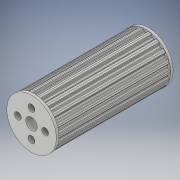
# Autodesk Inventor part: Pulley
Saved by Autodesk Inventor 2019 (Build 230136000, 136)
## iProperties
Created: 2019-03-22
Part Number: Pulley
Material: Generic
Document SubType Name: Modeling
Designer: frown
Density: 1 g/cm^3
Appearance: Default
Author: frown
Autodesk Inventor part; units mm, degrees
ref_plane "YZ Plane" through (0, 0, 0) normal (1, 0, 0) x (0, 1, 0)
ref_plane "XZ Plane" through (0, 0, 0) normal (0, 1, 0) x (-1, 0, 0)
ref_plane "XY Plane" through (0, 0, 0) normal (0, 0, 1) x (1, 0, 0)
sketch "Sketch1" plane through (-11.8161, 5.8463, 20) normal (0, 0, 1) x (1, 0, 0)
  circle A0 centre (11.8162, -5.8464) radius 2.6001 projected
  line L0 (0.3323, 2.2358) -> (0.845, 1.4636) construction
  line L1 (2.7121, 3.6888) -> (1.8626, 4.0596)
  line L2 (0.8623, 3.345) -> (1.4764, 4.0152)
  line L3 (0.8623, 3.345) -> (0.309, 2.6238)
  line L4 (0.3323, 2.2358) -> (0.845, 1.4636)
  line L5 (3.8664, 4.3699) -> (3.1355, 3.7567)
  arc A1 (1.8626, 4.0596) -> (1.4764, 4.0152) centre (1.7083, 3.7) ccw
  arc A2 (2.7121, 3.6888) -> (3.1355, 3.7567) centre (2.8686, 4.0672) ccw
  arc A3 (0.309, 2.6238) -> (0.3323, 2.2358) centre (0.6547, 2.4499) ccw
  arc A4 (0.8516, 1.0348) -> (0.845, 1.4636) centre (0.4997, 1.2438) ccw
  arc A5 (-0.8406, -3.1302) -> (-0.9935, -2.7296) centre (-1.2428, -3.0542) ccw
  line L6 (-1.7394, -2.1793) -> (-0.9935, -2.7296)
  line L7 (0, 0) -> (-0.9251, 0.0579)
  arc A6 (-1.894, -1.8227) -> (-1.7394, -2.1793) centre (-1.5096, -1.8679) ccw
  arc A7 (-0.9251, 0.0579) -> (-1.2729, -0.1159) centre (-0.9471, -0.3328) ccw
  line L8 (-1.6207, -0.9557) -> (-1.894, -1.8227)
  line L9 (-1.6207, -0.9557) -> (-1.2729, -0.1159)
  arc A8 (-1.0063, -7.6229) -> (-1.287, -7.2987) centre (-1.4102, -7.689) ccw
  line L10 (-0.8406, -3.1302) -> (-1.0063, -4.0697)
  arc A9 (-1.287, -4.3939) -> (-1.0063, -4.0697) centre (-1.4103, -4.0035) ccw
  line L11 (-2.1761, -7.0367) -> (-1.287, -7.2987)
  line L12 (-1.287, -4.3939) -> (-2.1761, -4.6559)
  arc A10 (-2.4433, -6.7544) -> (-2.1761, -7.0367) centre (-2.0667, -6.6655) ccw
  arc A11 (-2.1761, -4.6559) -> (-2.4434, -4.9382) centre (-2.0631, -5.0306) ccw
  line L13 (-2.4831, -5.8463) -> (-2.4433, -6.7544)
  line L14 (-2.4831, -5.8463) -> (-2.4434, -4.9382)
  arc A12 (0.3746, -11.9013) -> (0, -11.6926) centre (0.0177, -12.1015) ccw
  line L15 (-1.0063, -7.6229) -> (-0.8406, -8.5624)
  arc A13 (-0.9935, -8.963) -> (-0.8406, -8.5624) centre (-1.243, -8.6384) ccw
  line L16 (-0.9251, -11.7505) -> (0, -11.6926)
  line L17 (-0.9935, -8.963) -> (-1.7394, -9.5133)
  arc A14 (-1.2728, -11.5767) -> (-0.9251, -11.7505) centre (-0.9493, -11.3643) ccw
  arc A15 (-1.7394, -9.5133) -> (-1.8941, -9.87) centre (-1.5051, -9.8268) ccw
  line L18 (-1.6207, -10.7369) -> (-1.2728, -11.5767)
  line L19 (-1.6207, -10.7369) -> (-1.8941, -9.87)
  arc A16 (3.1356, -15.4493) -> (2.7121, -15.3814) centre (2.8686, -15.7595) ccw
  line L20 (0.3746, -11.9013) -> (0.8516, -12.7274)
  arc A17 (0.845, -13.1562) -> (0.8516, -12.7274) centre (0.4995, -12.9364) ccw
  line L21 (1.8627, -15.7522) -> (2.7121, -15.3814)
  line L22 (0.845, -13.1562) -> (0.3323, -13.9284)
  arc A18 (1.4765, -15.7078) -> (1.8627, -15.7522) centre (1.7078, -15.3975) ccw
  arc A19 (0.3323, -13.9284) -> (0.309, -14.3165) centre (0.6597, -14.1428) ccw
  line L23 (0.8623, -15.0376) -> (1.4765, -15.7078)
  line L24 (0.8623, -15.0376) -> (0.309, -14.3165)
  arc A20 (6.9435, -17.8391) -> (6.5224, -17.9201) centre (6.7988, -18.2219) ccw
  line L25 (3.1356, -15.4493) -> (3.8663, -16.0625)
  arc A21 (4.0068, -16.4677) -> (3.8663, -16.0625) centre (3.607, -16.3793) ccw
  line L26 (5.8509, -18.5591) -> (6.5224, -17.9201)
  line L27 (4.0068, -16.4677) -> (3.7891, -17.3687)
  arc A22 (5.4728, -18.6494) -> (5.8509, -18.5591) centre (5.5841, -18.2787) ccw
  arc A23 (3.7891, -17.3687) -> (3.8999, -17.7413) centre (4.1701, -17.4582) ccw
  line L28 (4.6665, -18.2297) -> (5.4728, -18.6494)
  line L29 (4.6665, -18.2297) -> (3.8999, -17.7413)
  arc A24 (11.3391, -18.7824) -> (10.9711, -19.0025) centre (11.3341, -19.1916) ccw
  line L30 (6.9435, -17.8391) -> (7.8399, -18.1654)
  arc A25 (8.1105, -18.4981) -> (7.8399, -18.1654) centre (7.7046, -18.5518) ccw
  line L31 (10.5587, -19.8326) -> (10.9711, -19.0025)
  line L32 (8.1105, -18.4981) -> (8.2141, -19.4192)
  arc A26 (10.2343, -20.0468) -> (10.5587, -19.8326) centre (10.2121, -19.6604) ccw
  arc A27 (8.2141, -19.4192) -> (8.4456, -19.7315) centre (8.6027, -19.373) ccw
  line L33 (9.3331, -19.9282) -> (10.2343, -20.0468)
  line L34 (9.3331, -19.9282) -> (8.4456, -19.7315)
  arc A28 (15.7923, -18.1654) -> (15.5217, -18.4981) centre (15.9275, -18.5517) ccw
  line L35 (11.3391, -18.7824) -> (12.2931, -18.7824)
  arc A29 (12.6611, -19.0025) -> (12.2931, -18.7824) centre (12.2981, -19.1918) ccw
  line L36 (15.4181, -19.4192) -> (15.5217, -18.4981)
  line L37 (12.6611, -19.0025) -> (13.0735, -19.8326)
  arc A30 (15.1866, -19.7314) -> (15.4181, -19.4192) centre (15.0335, -19.3759) ccw
  arc A31 (13.0735, -19.8326) -> (13.3979, -20.0469) centre (13.4229, -19.6563) ccw
  line L38 (14.2991, -19.9282) -> (15.1866, -19.7314)
  line L39 (14.2991, -19.9282) -> (13.3979, -20.0469)
  arc A32 (19.7658, -16.0625) -> (19.6254, -16.4677) centre (20.025, -16.3793) ccw
  line L40 (15.7923, -18.1654) -> (16.6887, -17.8391)
  arc A33 (17.1098, -17.9201) -> (16.6887, -17.8391) centre (16.8334, -18.2221) ccw
  line L41 (19.8431, -17.3687) -> (19.6254, -16.4677)
  line L42 (17.1098, -17.9201) -> (17.7813, -18.5591)
  arc A34 (19.7323, -17.7413) -> (19.8431, -17.3687) centre (19.4669, -17.4596) ccw
  arc A35 (17.7813, -18.5591) -> (18.1594, -18.6495) centre (18.0493, -18.2739) ccw
  line L43 (18.9657, -18.2297) -> (19.7323, -17.7413)
  line L44 (18.9657, -18.2297) -> (18.1594, -18.6495)
  arc A36 (22.7806, -12.7274) -> (22.7872, -13.1562) centre (23.1325, -12.9364) ccw
  line L45 (19.7658, -16.0625) -> (20.4967, -15.4493)
  arc A37 (20.9201, -15.3814) -> (20.4967, -15.4493) centre (20.7636, -15.7598) ccw
  line L46 (23.2999, -13.9284) -> (22.7872, -13.1562)
  line L47 (20.9201, -15.3814) -> (21.7695, -15.7522)
  arc A38 (23.3232, -14.3164) -> (23.2999, -13.9284) centre (22.9775, -14.1425) ccw
  arc A39 (21.7695, -15.7522) -> (22.1558, -15.7078) centre (21.9239, -15.3926) ccw
  line L48 (22.7699, -15.0376) -> (23.3232, -14.3164)
  line L49 (22.7699, -15.0376) -> (22.1558, -15.7078)
  arc A40 (24.4728, -8.5624) -> (24.6257, -8.963) centre (24.875, -8.6384) ccw
  line L50 (22.7806, -12.7274) -> (23.2576, -11.9012)
  arc A41 (23.6322, -11.6926) -> (23.2576, -11.9012) centre (23.6146, -12.1017) ccw
  line L51 (25.3716, -9.5133) -> (24.6257, -8.963)
  line L52 (23.6322, -11.6926) -> (24.5573, -11.7505)
  arc A42 (25.5262, -9.8699) -> (25.3716, -9.5133) centre (25.1418, -9.8247) ccw
  arc A43 (24.5573, -11.7505) -> (24.9051, -11.5767) centre (24.5793, -11.3598) ccw
  line L53 (25.2529, -10.7369) -> (25.5262, -9.8699)
  line L54 (25.2529, -10.7369) -> (24.9051, -11.5767)
  arc A44 (24.6385, -4.0697) -> (24.9192, -4.3939) centre (25.0424, -4.0036) ccw
  line L55 (24.4728, -8.5624) -> (24.6385, -7.6229)
  arc A45 (24.9192, -7.2987) -> (24.6385, -7.6229) centre (25.0425, -7.6891) ccw
  line L56 (25.8083, -4.6559) -> (24.9192, -4.3939)
  line L57 (24.9192, -7.2987) -> (25.8083, -7.0367)
  arc A46 (26.0755, -4.9382) -> (25.8083, -4.6559) centre (25.6989, -5.0271) ccw
  arc A47 (25.8083, -7.0367) -> (26.0756, -6.7544) centre (25.6953, -6.662) ccw
  line L58 (26.1153, -5.8463) -> (26.0755, -4.9382)
  line L59 (26.1153, -5.8463) -> (26.0756, -6.7544)
  arc A48 (23.2576, 0.2087) -> (23.6322, 0) centre (23.6145, 0.4089) ccw
  line L60 (24.6385, -4.0697) -> (24.4728, -3.1302)
  arc A49 (24.6257, -2.7296) -> (24.4728, -3.1302) centre (24.8752, -3.0542) ccw
  line L61 (24.5573, 0.0579) -> (23.6322, 0)
  line L62 (24.6257, -2.7296) -> (25.3716, -2.1793)
  arc A50 (24.905, -0.1159) -> (24.5573, 0.0579) centre (24.5815, -0.3283) ccw
  arc A51 (25.3716, -2.1793) -> (25.5263, -1.8226) centre (25.1373, -1.8658) ccw
  line L63 (25.2529, -0.9557) -> (24.905, -0.1159)
  line L64 (25.2529, -0.9557) -> (25.5263, -1.8226)
  arc A52 (20.4966, 3.7567) -> (20.9201, 3.6888) centre (20.7636, 4.0669) ccw
  line L65 (23.2576, 0.2087) -> (22.7806, 1.0348)
  arc A53 (22.7872, 1.4636) -> (22.7806, 1.0348) centre (23.1327, 1.2438) ccw
  line L66 (21.7695, 4.0596) -> (20.9201, 3.6888)
  line L67 (22.7872, 1.4636) -> (23.2999, 2.2358)
  arc A54 (22.1557, 4.0152) -> (21.7695, 4.0596) centre (21.9244, 3.7049) ccw
  arc A55 (23.2999, 2.2358) -> (23.3232, 2.6239) centre (22.9725, 2.4502) ccw
  line L68 (22.7699, 3.345) -> (22.1557, 4.0152)
  line L69 (22.7699, 3.345) -> (23.3232, 2.6239)
  arc A56 (16.6887, 6.1465) -> (17.1098, 6.2275) centre (16.8334, 6.5293) ccw
  line L70 (20.4966, 3.7567) -> (19.7659, 4.3699)
  arc A57 (19.6254, 4.7751) -> (19.7659, 4.3699) centre (20.0252, 4.6867) ccw
  line L71 (17.7813, 6.8665) -> (17.1098, 6.2275)
  line L72 (19.6254, 4.7751) -> (19.8431, 5.6761)
  arc A58 (18.1594, 6.9568) -> (17.7813, 6.8665) centre (18.0481, 6.5861) ccw
  arc A59 (19.8431, 5.6761) -> (19.7323, 6.0487) centre (19.4621, 5.7656) ccw
  line L73 (18.9657, 6.5371) -> (18.1594, 6.9568)
  line L74 (18.9657, 6.5371) -> (19.7323, 6.0487)
  arc A60 (12.2931, 7.0898) -> (12.6611, 7.3099) centre (12.2981, 7.499) ccw
  line L75 (16.6887, 6.1465) -> (15.7923, 6.4728)
  arc A61 (15.5217, 6.8055) -> (15.7923, 6.4728) centre (15.9276, 6.8592) ccw
  line L76 (13.0735, 8.14) -> (12.6611, 7.3099)
  line L77 (15.5217, 6.8055) -> (15.4181, 7.7266)
  arc A62 (13.3979, 8.3542) -> (13.0735, 8.14) centre (13.4201, 7.9678) ccw
  arc A63 (15.4181, 7.7266) -> (15.1866, 8.0389) centre (15.0295, 7.6804) ccw
  line L78 (14.2991, 8.2356) -> (13.3979, 8.3542)
  line L79 (14.2991, 8.2356) -> (15.1866, 8.0389)
  arc A64 (7.8399, 6.4728) -> (8.1105, 6.8055) centre (7.7047, 6.8591) ccw
  line L80 (12.2931, 7.0898) -> (11.3391, 7.0898)
  arc A65 (10.9711, 7.3099) -> (11.3391, 7.0898) centre (11.3341, 7.4992) ccw
  line L81 (8.2141, 7.7266) -> (8.1105, 6.8055)
  line L82 (10.9711, 7.3099) -> (10.5587, 8.14)
  arc A66 (8.4456, 8.0388) -> (8.2141, 7.7266) centre (8.5987, 7.6833) ccw
  arc A67 (10.5587, 8.14) -> (10.2343, 8.3543) centre (10.2093, 7.9637) ccw
  line L83 (9.3331, 8.2356) -> (8.4456, 8.0388)
  line L84 (9.3331, 8.2356) -> (10.2343, 8.3543)
  arc A68 (3.8664, 4.3699) -> (4.0068, 4.7751) centre (3.6072, 4.6867) ccw
  line L85 (7.8399, 6.4728) -> (6.9435, 6.1465)
  arc A69 (6.5224, 6.2275) -> (6.9435, 6.1465) centre (6.7988, 6.5295) ccw
  line L86 (3.7891, 5.6761) -> (4.0068, 4.7751)
  line L87 (6.5224, 6.2275) -> (5.8509, 6.8665)
  arc A70 (3.8999, 6.0487) -> (3.7891, 5.6761) centre (4.1653, 5.767) ccw
  arc A71 (5.8509, 6.8665) -> (5.4728, 6.9569) centre (5.5829, 6.5813) ccw
  line L88 (4.6665, 6.5371) -> (3.8999, 6.0487)
  line L89 (4.6665, 6.5371) -> (5.4728, 6.9569)
  line L90 (0.8516, 1.0348) -> (0.3746, 0.2087)
  arc A72 (0, 0) -> (0.3746, 0.2087) centre (0.0176, 0.4092) ccw
  point P0 (11.8161, -5.8463)
  point P1 (0.2852, 2.3363)
  point P2 (2.819, 3.66)
  point P3 (2.9298, 3.6623)
  point P4 (1.6446, 4.0861)
  point P5 (0.9089, 1.2538)
  point P6 (20.4966, 3.7567)
  point P7 (16.6887, 6.1465)
  point P8 (12.2931, 7.0898)
  point P9 (7.8399, 6.4728)
  point P10 (-0.8617, -2.9048)
  point P11 (0.2136, 0.0496)
  point P12 (-1.1391, 0.0082)
  point P13 (-1.1032, -7.4183)
  point P14 (-1.1032, -4.2743)
  point P15 (-2.3601, -4.7758)
  point P16 (0.2136, -11.7421)
  point P17 (-0.8617, -8.7877)
  point P18 (-1.8714, -9.6889)
  point P19 (2.9298, -15.3549)
  point P20 (0.9089, -12.9464)
  point P21 (0.2683, -14.1385)
  point P22 (6.7179, -17.8207)
  point P23 (3.995, -16.2487)
  point P24 (3.8009, -17.588)
  point P25 (11.1208, -18.8423)
  point P26 (8.0245, -18.2964)
  point P27 (8.3001, -19.6213)
  point P28 (15.6076, -18.2963)
  point P29 (12.5114, -18.8423)
  point P30 (13.2235, -19.9931)
  point P31 (19.6371, -16.2487)
  point P32 (16.9143, -17.8208)
  point P33 (17.9771, -18.6586)
  point P34 (22.7233, -12.9464)
  point P35 (20.7024, -15.3549)
  point P36 (21.9876, -15.7787)
  point P37 (24.4939, -8.7878)
  point P38 (23.4186, -11.7422)
  point P39 (24.7713, -11.7008)
  point P40 (24.7354, -4.2743)
  point P41 (24.7354, -7.4183)
  point P42 (25.9923, -6.9168)
  point P43 (23.4186, 0.0495)
  point P44 (24.4939, -2.9049)
  point P45 (25.5036, -2.0037)
  point P46 (20.7024, 3.6623)
  point P47 (22.7233, 1.2538)
  point P48 (23.3639, 2.4459)
  point P49 (16.9143, 6.1281)
  point P50 (19.6372, 4.5561)
  point P51 (19.8313, 5.8954)
  point P52 (20.4966, 3.7567)
  point P53 (12.5114, 7.1497)
  point P54 (15.6077, 6.6038)
  point P55 (15.3321, 7.9287)
  point P56 (16.6887, 6.1465)
  point P57 (8.0246, 6.6037)
  point P58 (11.1208, 7.1497)
  point P59 (10.4087, 8.3005)
  point P60 (12.2931, 7.0898)
  point P61 (3.9951, 4.5561)
  point P62 (6.7179, 6.1282)
  point P63 (5.6551, 6.966)
  point P64 (7.8399, 6.4728)
  dimension "d2" = 360
  constraints: 198 point on circle, 180 end point, 72 centre point, 34 coincident, 1 collinear, 1 tangent, 19 other
sketch "Sketch2" plane through (-11.8161, 5.8463, 20) normal (0, 0, 1) x (1, 0, 0)
  line L0 (0.8623, 3.345) -> (0.309, 2.6238) projected
  line L1 (1.4764, 4.0152) -> (0.8623, 3.345) projected
  line L2 (2.7121, 3.6888) -> (1.8626, 4.0596) projected
  line L3 (0.3323, 2.2358) -> (0.845, 1.4636) projected
  arc A0 (2.7121, 3.6888) -> (3.1355, 3.7567) centre (2.8686, 4.0672) ccw
  arc A1 (1.8626, 4.0596) -> (1.4764, 4.0152) centre (1.7083, 3.7) ccw
  arc A2 (0.309, 2.6238) -> (0.3323, 2.2358) centre (0.6591, 2.4501) ccw
  arc A3 (0.8516, 1.0348) -> (0.845, 1.4636) centre (0.4999, 1.2439) ccw
  line L4 (0.8516, 1.0348) -> (11.8161, -5.8463)
  line L5 (11.8161, -5.8463) -> (3.1355, 3.7567)
  point P0 (1.6446, 4.0861)
  point P1 (0.9089, 1.2538)
  point P2 (2.9298, 3.6623)
  point P3 (2.9298, 3.6623)
  point P4 (0.2683, 2.4458)
  point P5 (0.2683, 2.4458)
  constraints: 12 point on circle, 4 centre point, 4 end point, 2 coincident
extrude "Extrusion1" add sketch "Sketch2" along normal blind 0.125
pattern_circular "Circular Pattern1" count 18 over 360 about axis through (0, 0, 20) along (0, 0, 1) of "Extrusion1"
sketch "Sketch3" plane through (-11.8161, 5.8463, 20.125) normal (0, 0, 1) x (1, 0, 0)
  line L0 (11.8161, -5.8463) -> (3.1355, 3.7567) projected
  line L1 (3.8663, 4.3699) -> (11.8161, -5.8463) projected
  line L2 (3.1355, 3.7567) -> (3.8663, 4.3699)
  constraints: 2 end point
extrude "Extrusion2" add sketch "Sketch3" against normal blind 0.125
pattern_circular "Circular Pattern2" count 18 over 360 about axis through (0, 0, 20) along (0, 0, 1) of "Extrusion2"
sketch "Sketch4" plane through (-11.8161, 5.8463, 20.125) normal (0, 0, 1) x (1, 0, 0)
  arc A0 (6.5224, 6.2275) -> (6.9435, 6.1465) centre (6.7988, 6.5295) ccw projected
  line L0 (6.5224, 6.2275) -> (5.8509, 6.8665) projected
  arc A1 (5.8509, 6.8665) -> (5.4728, 6.9569) centre (5.5829, 6.5813) ccw projected
  line L1 (5.4728, 6.9569) -> (4.6665, 6.5371) projected
  line L2 (4.6665, 6.5371) -> (3.8999, 6.0487) projected
  arc A2 (3.8999, 6.0487) -> (3.7891, 5.6761) centre (4.1695, 5.7657) ccw projected
  line L3 (3.7891, 5.6761) -> (4.0068, 4.7751) projected
  arc A3 (3.8663, 4.3699) -> (4.0068, 4.7751) centre (3.6073, 4.6866) ccw projected
  line L4 (3.1355, 3.7567) -> (3.8663, 4.3699) projected
  arc A4 (2.7121, 3.6888) -> (3.1355, 3.7567) centre (2.8686, 4.0672) ccw projected
  line L5 (2.7121, 3.6888) -> (1.8626, 4.0596) projected
  arc A5 (1.8626, 4.0596) -> (1.4764, 4.0152) centre (1.7083, 3.7) ccw projected
  line L6 (1.4764, 4.0152) -> (0.8623, 3.345) projected
  line L7 (0.8623, 3.345) -> (0.309, 2.6238) projected
  arc A6 (0.309, 2.6238) -> (0.3323, 2.2358) centre (0.6591, 2.4501) ccw projected
  line L8 (0.3323, 2.2358) -> (0.845, 1.4636) projected
  arc A7 (0.8516, 1.0348) -> (0.845, 1.4636) centre (0.4999, 1.2439) ccw projected
  line L9 (0.3746, 0.2086) -> (0.8516, 1.0348) projected
  arc A8 (0, 0) -> (0.3746, 0.2086) centre (0.0176, 0.4091) ccw projected
  line L10 (0, 0) -> (-0.9251, 0.0579) projected
  arc A9 (-0.9251, 0.0579) -> (-1.2729, -0.1159) centre (-0.9471, -0.3328) ccw projected
  line L11 (-1.2729, -0.1159) -> (-1.6207, -0.9557) projected
  line L12 (-1.6207, -0.9557) -> (-1.894, -1.8227) projected
  arc A10 (-1.894, -1.8227) -> (-1.7394, -2.1793) centre (-1.5056, -1.8661) ccw projected
  line L13 (-1.7394, -2.1793) -> (-0.9935, -2.7296) projected
  arc A11 (-0.8407, -3.1302) -> (-0.9935, -2.7296) centre (-1.2426, -3.0541) ccw projected
  line L14 (-1.0063, -4.0697) -> (-0.8407, -3.1302) projected
  arc A12 (-1.287, -4.3939) -> (-1.0063, -4.0697) centre (-1.4103, -4.0035) ccw projected
  line L15 (-1.287, -4.3939) -> (-2.1761, -4.6559) projected
  arc A13 (-2.1761, -4.6559) -> (-2.4434, -4.9382) centre (-2.0631, -5.0306) ccw projected
  line L16 (-2.4434, -4.9382) -> (-2.4831, -5.8463) projected
  line L17 (-2.4831, -5.8463) -> (-2.4433, -6.7544) projected
  arc A14 (-2.4433, -6.7544) -> (-2.1761, -7.0367) centre (-2.0635, -6.6625) ccw projected
  line L18 (-2.1761, -7.0367) -> (-1.287, -7.2987) projected
  arc A15 (-1.0063, -7.6229) -> (-1.287, -7.2987) centre (-1.4101, -7.6888) ccw projected
  line L19 (-0.8406, -8.5624) -> (-1.0063, -7.6229) projected
  arc A16 (-0.9935, -8.963) -> (-0.8406, -8.5624) centre (-1.243, -8.6384) ccw projected
  line L20 (-0.9935, -8.963) -> (-1.7394, -9.5133) projected
  arc A17 (-1.7394, -9.5133) -> (-1.8941, -9.87) centre (-1.5051, -9.8268) ccw projected
  line L21 (-1.8941, -9.87) -> (-1.6207, -10.7369) projected
  line L22 (-1.6207, -10.7369) -> (-1.2728, -11.5767) projected
  arc A18 (-1.2728, -11.5767) -> (-0.9251, -11.7505) centre (-0.9473, -11.3604) ccw projected
  line L23 (-0.9251, -11.7505) -> (0, -11.6926) projected
  arc A19 (0.3746, -11.9013) -> (0, -11.6926) centre (0.0177, -12.1013) ccw projected
  line L24 (0.8516, -12.7274) -> (0.3746, -11.9013) projected
  arc A20 (0.845, -13.1562) -> (0.8516, -12.7274) centre (0.4995, -12.9364) ccw projected
  line L25 (0.845, -13.1562) -> (0.3323, -13.9284) projected
  arc A21 (0.3323, -13.9284) -> (0.309, -14.3165) centre (0.6597, -14.1428) ccw projected
  line L26 (0.309, -14.3165) -> (0.8623, -15.0376) projected
  line L27 (0.8623, -15.0376) -> (1.4765, -15.7078) projected
  arc A22 (1.4765, -15.7078) -> (1.8627, -15.7522) centre (1.7083, -15.3932) ccw projected
  line L28 (1.8627, -15.7522) -> (2.7121, -15.3814) projected
  arc A23 (3.1355, -15.4493) -> (2.7121, -15.3814) centre (2.8686, -15.7594) ccw projected
  line L29 (3.8663, -16.0625) -> (3.1355, -15.4493) projected
  arc A24 (4.0068, -16.4677) -> (3.8663, -16.0625) centre (3.607, -16.3793) ccw projected
  line L30 (4.0068, -16.4677) -> (3.7891, -17.3687) projected
  arc A25 (3.7891, -17.3687) -> (3.8999, -17.7413) centre (4.1701, -17.4582) ccw projected
  line L31 (3.8999, -17.7413) -> (4.6665, -18.2297) projected
  line L32 (4.6665, -18.2297) -> (5.4728, -18.6494) projected
  arc A26 (5.4728, -18.6494) -> (5.8509, -18.5591) centre (5.5831, -18.2745) ccw projected
  line L33 (5.8509, -18.5591) -> (6.5224, -17.9201) projected
  arc A27 (6.9435, -17.8391) -> (6.5224, -17.9201) centre (6.7987, -18.2218) ccw projected
  line L34 (7.8399, -18.1654) -> (6.9435, -17.8391) projected
  arc A28 (8.1105, -18.4981) -> (7.8399, -18.1654) centre (7.7046, -18.5518) ccw projected
  line L35 (8.1105, -18.4981) -> (8.2141, -19.4192) projected
  arc A29 (8.2141, -19.4192) -> (8.4456, -19.7315) centre (8.6027, -19.373) ccw projected
  line L36 (8.4456, -19.7315) -> (9.3331, -19.9282) projected
  line L37 (9.3331, -19.9282) -> (10.2343, -20.0468) projected
  arc A30 (10.2343, -20.0468) -> (10.5587, -19.8326) centre (10.2097, -19.6568) ccw projected
  line L38 (10.5587, -19.8326) -> (10.9711, -19.0025) projected
  arc A31 (11.3391, -18.7824) -> (10.9711, -19.0025) centre (11.3339, -19.1915) ccw projected
  line L39 (12.2931, -18.7824) -> (11.3391, -18.7824) projected
  arc A32 (12.6611, -19.0025) -> (12.2931, -18.7824) centre (12.2981, -19.1918) ccw projected
  line L40 (12.6611, -19.0025) -> (13.0735, -19.8326) projected
  arc A33 (13.0735, -19.8326) -> (13.3979, -20.0469) centre (13.4229, -19.6563) ccw projected
  line L41 (13.3979, -20.0469) -> (14.2991, -19.9282) projected
  line L42 (14.2991, -19.9282) -> (15.1866, -19.7314) projected
  arc A34 (15.1866, -19.7314) -> (15.4181, -19.4192) centre (15.0301, -19.3733) ccw projected
  line L43 (15.4181, -19.4192) -> (15.5217, -18.4981) projected
  arc A35 (15.7923, -18.1654) -> (15.5217, -18.4981) centre (15.9273, -18.5516) ccw projected
  line L44 (16.6887, -17.8391) -> (15.7923, -18.1654) projected
  arc A36 (17.1098, -17.9201) -> (16.6887, -17.8391) centre (16.8334, -18.2221) ccw projected
  line L45 (17.1098, -17.9201) -> (17.7813, -18.5591) projected
  arc A37 (17.7813, -18.5591) -> (18.1594, -18.6495) centre (18.0493, -18.2739) ccw projected
  line L46 (18.1594, -18.6495) -> (18.9657, -18.2297) projected
  line L47 (18.9657, -18.2297) -> (19.7323, -17.7413) projected
  arc A38 (19.7323, -17.7413) -> (19.8431, -17.3687) centre (19.4627, -17.4583) ccw projected
  line L48 (19.8431, -17.3687) -> (19.6254, -16.4677) projected
  arc A39 (19.7659, -16.0625) -> (19.6254, -16.4677) centre (20.0249, -16.3792) ccw projected
  line L49 (20.4967, -15.4493) -> (19.7659, -16.0625) projected
  arc A40 (20.9201, -15.3814) -> (20.4967, -15.4493) centre (20.7636, -15.7598) ccw projected
  line L50 (20.9201, -15.3814) -> (21.7695, -15.7522) projected
  arc A41 (21.7695, -15.7522) -> (22.1558, -15.7078) centre (21.9239, -15.3926) ccw projected
  line L51 (22.1558, -15.7078) -> (22.7699, -15.0376) projected
  line L52 (22.7699, -15.0376) -> (23.3232, -14.3164) projected
  arc A42 (23.3232, -14.3164) -> (23.2999, -13.9284) centre (22.9731, -14.1427) ccw projected
  line L53 (23.2999, -13.9284) -> (22.7872, -13.1562) projected
  arc A43 (22.7806, -12.7275) -> (22.7872, -13.1562) centre (23.1323, -12.9365) ccw projected
  line L54 (23.2576, -11.9012) -> (22.7806, -12.7275) projected
  arc A44 (23.6322, -11.6926) -> (23.2576, -11.9012) centre (23.6146, -12.1017) ccw projected
  line L55 (23.6322, -11.6926) -> (24.5573, -11.7505) projected
  arc A45 (24.5573, -11.7505) -> (24.9051, -11.5767) centre (24.5793, -11.3598) ccw projected
  line L56 (24.9051, -11.5767) -> (25.2529, -10.7369) projected
  line L57 (25.2529, -10.7369) -> (25.5262, -9.8699) projected
  arc A46 (25.5262, -9.8699) -> (25.3716, -9.5133) centre (25.1378, -9.8265) ccw projected
  line L58 (25.3716, -9.5133) -> (24.6257, -8.963) projected
  arc A47 (24.4729, -8.5624) -> (24.6257, -8.963) centre (24.8748, -8.6385) ccw projected
  line L59 (24.6385, -7.6229) -> (24.4729, -8.5624) projected
  arc A48 (24.9192, -7.2987) -> (24.6385, -7.6229) centre (25.0425, -7.6891) ccw projected
  line L60 (24.9192, -7.2987) -> (25.8083, -7.0367) projected
  arc A49 (25.8083, -7.0367) -> (26.0756, -6.7544) centre (25.6953, -6.662) ccw projected
  line L61 (26.0756, -6.7544) -> (26.1153, -5.8463) projected
  line L62 (26.1153, -5.8463) -> (26.0755, -4.9382) projected
  arc A50 (26.0755, -4.9382) -> (25.8083, -4.6559) centre (25.6957, -5.0301) ccw projected
  line L63 (25.8083, -4.6559) -> (24.9192, -4.3939) projected
  arc A51 (24.6385, -4.0697) -> (24.9192, -4.3939) centre (25.0423, -4.0038) ccw projected
  line L64 (24.4728, -3.1302) -> (24.6385, -4.0697) projected
  arc A52 (24.6257, -2.7296) -> (24.4728, -3.1302) centre (24.8752, -3.0542) ccw projected
  line L65 (24.6257, -2.7296) -> (25.3716, -2.1793) projected
  arc A53 (25.3716, -2.1793) -> (25.5263, -1.8226) centre (25.1373, -1.8658) ccw projected
  line L66 (25.5263, -1.8226) -> (25.2529, -0.9557) projected
  line L67 (25.2529, -0.9557) -> (24.905, -0.1159) projected
  arc A54 (24.905, -0.1159) -> (24.5573, 0.0579) centre (24.5795, -0.3322) ccw projected
  line L68 (24.5573, 0.0579) -> (23.6322, 0) projected
  arc A55 (23.2576, 0.2087) -> (23.6322, 0) centre (23.6145, 0.4087) ccw projected
  line L69 (22.7806, 1.0348) -> (23.2576, 0.2087) projected
  arc A56 (22.7872, 1.4636) -> (22.7806, 1.0348) centre (23.1327, 1.2438) ccw projected
  line L70 (22.7872, 1.4636) -> (23.2999, 2.2358) projected
  arc A57 (23.2999, 2.2358) -> (23.3232, 2.6239) centre (22.9725, 2.4502) ccw projected
  line L71 (23.3232, 2.6239) -> (22.7699, 3.345) projected
  line L72 (22.7699, 3.345) -> (22.1557, 4.0152) projected
  arc A58 (22.1557, 4.0152) -> (21.7695, 4.0596) centre (21.9239, 3.7006) ccw projected
  line L73 (21.7695, 4.0596) -> (20.9201, 3.6888) projected
  arc A59 (20.4967, 3.7567) -> (20.9201, 3.6888) centre (20.7636, 4.0668) ccw projected
  line L74 (19.7659, 4.3699) -> (20.4967, 3.7567) projected
  arc A60 (19.6254, 4.7751) -> (19.7659, 4.3699) centre (20.0252, 4.6867) ccw projected
  line L75 (19.6254, 4.7751) -> (19.8431, 5.6761) projected
  arc A61 (19.8431, 5.6761) -> (19.7323, 6.0487) centre (19.4621, 5.7656) ccw projected
  line L76 (19.7323, 6.0487) -> (18.9657, 6.5371) projected
  line L77 (18.9657, 6.5371) -> (18.1594, 6.9568) projected
  arc A62 (18.1594, 6.9568) -> (17.7813, 6.8665) centre (18.0491, 6.5819) ccw projected
  line L78 (17.7813, 6.8665) -> (17.1098, 6.2275) projected
  arc A63 (16.6887, 6.1465) -> (17.1098, 6.2275) centre (16.8335, 6.5292) ccw projected
  line L79 (15.7923, 6.4728) -> (16.6887, 6.1465) projected
  arc A64 (15.5217, 6.8055) -> (15.7923, 6.4728) centre (15.9276, 6.8592) ccw projected
  line L80 (15.5217, 6.8055) -> (15.4181, 7.7266) projected
  arc A65 (15.4181, 7.7266) -> (15.1866, 8.0389) centre (15.0295, 7.6804) ccw projected
  line L81 (15.1866, 8.0389) -> (14.2991, 8.2356) projected
  line L82 (14.2991, 8.2356) -> (13.3979, 8.3542) projected
  arc A66 (13.3979, 8.3542) -> (13.0735, 8.14) centre (13.4225, 7.9642) ccw projected
  line L83 (13.0735, 8.14) -> (12.6611, 7.3099) projected
  arc A67 (12.2931, 7.0898) -> (12.6611, 7.3099) centre (12.2983, 7.4989) ccw projected
  line L84 (11.3391, 7.0898) -> (12.2931, 7.0898) projected
  arc A68 (10.9711, 7.3099) -> (11.3391, 7.0898) centre (11.3341, 7.4992) ccw projected
  line L85 (10.9711, 7.3099) -> (10.5587, 8.14) projected
  arc A69 (10.5587, 8.14) -> (10.2343, 8.3543) centre (10.2093, 7.9637) ccw projected
  line L86 (10.2343, 8.3543) -> (9.3331, 8.2356) projected
  line L87 (9.3331, 8.2356) -> (8.4456, 8.0388) projected
  arc A70 (8.4456, 8.0388) -> (8.2141, 7.7266) centre (8.6021, 7.6807) ccw projected
  line L88 (8.2141, 7.7266) -> (8.1105, 6.8055) projected
  arc A71 (7.8399, 6.4728) -> (8.1105, 6.8055) centre (7.7049, 6.859) ccw projected
  line L89 (6.9435, 6.1465) -> (7.8399, 6.4728) projected
  point P0 (11.8161, -5.8463)
extrude "Extrusion3" add sketch "Sketch4" along normal blind 34.1313
sketch "Sketch5" plane through (-11.8161, 5.8463, 20) normal (0, 0, -1) x (-1, 0, 0)
  circle A0 centre (-11.8161, -5.8463) radius 14.5
  dimension "d20" = 29
  constraints: 1 centre point, 1 coincident
  measures "d20" diameter of A0
extrude "Extrusion4" add sketch "Sketch5" against normal blind 1.5875
mirror "Mirror1" about plane through (0, 0, 54.2563) normal (0, 0, 1)
sketch "Sketch6" plane through (0, 0, 88.5125) normal (0, 0, 1) x (1, 0, 0)
  line L0 (1.4434, 2.5) -> (2.8868, 0)
  line L1 (2.8868, 0) -> (1.4434, -2.5)
  line L2 (1.4434, -2.5) -> (-1.4434, -2.5)
  line L3 (-1.4434, -2.5) -> (-2.8868, 0)
  line L4 (-2.8868, 0) -> (-1.4434, 2.5)
  line L5 (-1.4434, 2.5) -> (1.4434, 2.5)
  circle A0 centre (0, 0) radius 3.3868
  circle A1 centre (0, 8) radius 2
  circle A2 centre (-8, 0) radius 2
  circle A3 centre (0, -8) radius 2
  circle A4 centre (8, 0) radius 2
  dimension "d23" = 2.5
  dimension "d24" = 6.7735
  dimension "d25" = 4
  dimension "d26" = 8
  dimension "d29" = 360
  constraints: 12 end point, 5 centre point, 2 coincident, 22 other
  measures "d23" distance from line of point (0, 0) L5
  measures "d24" diameter of A0
  measures "d25" diameter of A1
  measures "d26" distance of point (0, 0) A1.centre
extrude "Extrusion5" cut sketch "Sketch6" against normal through all contours L0 L1 L2 L3 L4 L5 | A0 | A1 | A2 | A3 | A4
body "Solid1"
